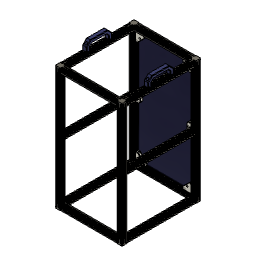
assembly (Autodesk Fusion 360 design; units mm, degrees)
Autodesk Fusion 360 part; units mm, degrees
sketch "Sketch1" plane through (0, 0, 0) normal (0, 0, 1) x (1, 0, 0) in component "2020-angle-connector"
  line L0 (10, 10) -> (-10, 10)
  line L1 (-10, 10) -> (-10, -10)
  line L2 (-10, -10) -> (10, -10)
  line L3 (10, -10) -> (10, 10)
  line L4 (10, 10) -> (-10, -10) construction
  line L5 (-10, 10) -> (10, -10) construction
  dimension "d1" = 20
  dimension "d2" = 20
  constraint horizontal L0
  constraint perpendicular L0 L1
  constraint parallel L0 L2
  constraint parallel L1 L3
  constraint coincident L4 origin
  constraint coincident L5 origin
  measures "d1" distance of L1.end L2.end
  measures "d2" distance of L0.end L1.end
extrude "Extrude1" add sketch "Sketch1" along normal blind 5 makes body 1 in component "2020-angle-connector"
fillet "Fillet1" radius 1.5 4 edges at (10, -10, 2.5) (-10, -10, 2.5) (10, 10, 2.5) (-10, 10, 2.5) on bodies 1 in component "2020-angle-connector"
sketch "Sketch2" plane through (0, -10, 0) normal (0, -1, 0) x (1, 0, 0) in component "2020-angle-connector"
  line L0 (-8.5, 5) -> (-8.5, 0)
  line L1 (-8.5, 0) -> (8.5, 0)
  line L2 (8.5, 0) -> (8.5, 5)
  line L3 (8.5, 5) -> (-8.5, 5)
  line L4 (-3, 5) -> (3, 5)
  line L5 (3, 5) -> (5, 3)
  line L6 (5, 3) -> (5, 1.5)
  line L7 (5, 1.5) -> (3, 1.5)
  line L8 (3, 1.5) -> (3, 0)
  line L9 (3, 0) -> (-3, 0)
  line L10 (-3, 0) -> (-3, 1.5)
  line L11 (-3, 1.5) -> (-5, 1.5)
  line L12 (-5, 1.5) -> (-5, 3)
  line L13 (-5, 3) -> (-3, 5)
  dimension "d7" = 10
  dimension "d8" = 6
  dimension "d9" = 135
  dimension "d11" = 1.5
  dimension "d12" = 6
  constraint parallel L3 L4
  constraint perpendicular L4 L6
  constraint perpendicular L6 L7
  constraint coincident L1 L8.end
  constraint perpendicular L1 L8
  constraint coincident L1 L9.end
  constraint perpendicular L9 L10
  constraint perpendicular L10 L11
  constraint perpendicular L11 L12
  constraint midpoint origin L9
  constraint midpoint L3 L4
  constraint equal L5 L13
  constraint equal L6 L12
  constraint equal L7 L11
  constraint equal L8 L10
  measures "d7" distance of L6 L12
  measures "d8" distance of L8 L10
  measures "d9" angle of L12 L13
  measures "d11" distance of L9.end L11
  measures "d12" distance of L4.start L4.end
extrude "Extrude2" add sketch "Sketch2" along normal blind 15.5 contours L1 L3 L4 L5 L6 L7 L8 L9 L10 L11 L12 L13 bodies 1 in component "2020-angle-connector"
pattern_circular "C-Pattern1" count 2 over 90 about axis through (0, 0, 1.75) along (0, 0, 1) of "Extrude2" in component "2020-angle-connector"
sketch "Sketch3" plane through (0, 0, 5) normal (0, 0, 1) x (-1, 0, 0) in component "2020-angle-connector"
  arc A0 (8.5, -10) -> (10, -8.5) centre (8.5, -8.5) ccw
  line L0 (10, -8.5) -> (10, 8.5)
  arc A1 (10, 8.5) -> (8.5, 10) centre (8.5, 8.5) ccw
  line L1 (8.5, 10) -> (3, 10)
  line L2 (3, 10) -> (3, 25.5)
  line L3 (3, 25.5) -> (-3, 25.5)
  line L4 (-3, 25.5) -> (-3, 10)
  line L5 (-3, 10) -> (-8.5, 10)
  arc A2 (-8.5, 10) -> (-10, 8.5) centre (-8.5, 8.5) ccw
  line L6 (-10, 8.5) -> (-10, 3)
  line L7 (-10, 3) -> (-25.5, 3)
  line L8 (-25.5, 3) -> (-25.5, -3)
  line L9 (-25.5, -3) -> (-10, -3)
  line L10 (-10, -3) -> (-10, -8.5)
  arc A3 (-10, -8.5) -> (-8.5, -10) centre (-8.5, -8.5) ccw
  line L11 (-8.5, -10) -> (8.5, -10)
  line L12 (10, -3) -> (10, 3)
  line L13 (10, 3) -> (8.5, 3)
  line L14 (8.5, 3) -> (8.5, 5)
  line L15 (8.5, 5) -> (7, 5)
  line L16 (7, 5) -> (5, 3)
  line L17 (5, 3) -> (5, -3)
  line L18 (5, -3) -> (7, -5)
  line L19 (7, -5) -> (8.5, -5)
  line L20 (8.5, -5) -> (8.5, -3)
  line L21 (8.5, -3) -> (10, -3)
  line L22 (5, 0) -> (10, 0) construction
  dimension "d17" = 6
  dimension "d18" = 10
  dimension "d19" = 1.5
  dimension "d20" = 5
  dimension "d21" = 6
  constraint coincident L0 L12.start
  constraint coincident L0 L12.end
  constraint perpendicular L0 L13
  constraint perpendicular L13 L14
  constraint perpendicular L14 L15
  constraint perpendicular L15 L17
  constraint perpendicular L16 L18
  constraint perpendicular L17 L19
  constraint perpendicular L19 L20
  constraint horizontal L21
  constraint equal L13 L21
  constraint equal L14 L20
  constraint equal L15 L19
  constraint equal L16 L18
  constraint midpoint L17 L22.start
  constraint midpoint L12 L22.end
  constraint midpoint L0 L12
  measures "d17" distance of L12.start L12.end
  measures "d18" distance of L15 L19
  measures "d19" distance of L12.start L20.end
  measures "d20" distance of L12 L17
  measures "d21" distance of L16.end L17.end
extrude "Extrude3" add sketch "Sketch3" along normal blind 15.5 contours L0 L12 L13 L14 L15 L16 L17 L18 L19 L20 L21 bodies 1 in component "2020-angle-connector"
pattern_circular "C-Pattern2" count 2 over 90 about axis through (0, 0, 1.75) along (0, 0, -1) of "Extrude3" in component "2020-angle-connector"
sketch "Sketch1 (2)" plane through (0, 0, 0) normal (0, 0, 1) x (1, 0, 0) in component "2020-profile-222,25"
  line L0 (-4.5, 0) -> (-4.5, 3.4393)
  line L1 (-7.0607, 6) -> (-8.5, 6)
  line L2 (-8.5, 6) -> (-8.5, 3)
  line L3 (-8.5, 3) -> (-10, 3)
  line L4 (-10, 3) -> (-10, 8.5)
  arc A0 (-8.5, 10) -> (-10, 8.5) centre (-8.5, 8.5) ccw
  line L5 (-8.5, 10) -> (-3, 10)
  line L6 (-3, 10) -> (-3, 8.5)
  line L7 (-3, 8.5) -> (-6, 8.5)
  line L8 (-6, 8.5) -> (-6, 7.0607)
  line L9 (-3.4393, 4.5) -> (0, 4.5)
  line L10 (0, 4.5) -> (0, 0)
  line L11 (0, 0) -> (-4.5, 0)
  line L12 (-7.0607, 6) -> (-4.5, 3.4393)
  line L13 (-6, 7.0607) -> (-3.4393, 4.5)
  circle A1 centre (0, 0) radius 2.75
  dimension "d26" = 10
  dimension "d27" = 1.5
  dimension "d28" = 4
  dimension "d29" = 5.5
  dimension "d30" = 10
  dimension "d31" = 6
  dimension "d33" = 1.5
  dimension "d34" = 3
  dimension "d35" = 5.5
  constraint vertical L0
  constraint perpendicular L0 L1
  constraint perpendicular L1 L2
  constraint perpendicular L0 L3
  constraint perpendicular L3 L4
  constraint tangent L4 A0
  constraint tangent A0 L5
  constraint perpendicular L4 L5
  constraint perpendicular L3 L6
  constraint perpendicular L6 L7
  constraint perpendicular L7 L8
  constraint perpendicular L8 L9
  constraint equal L1 L8
  constraint equal L2 L7
  constraint equal L3 L6
  constraint equal L4 L5
  constraint equal L0 L9
  constraint coincident L10.end L11.start
  constraint perpendicular L9 L10
  constraint horizontal L11
  constraint parallel L12 L13
  constraint equal L10 L11
  measures "d26" distance of L4 L10
  measures "d27" radius of A0
  measures "d28" distance of L0 L2
  measures "d29" distance of L0 L4
  measures "d30" distance of L10.end L5
  measures "d31" distance of L1 L11
  measures "d33" distance of L12 L13
  measures "d34" distance of L3 L11
  measures "d35" diameter of A1
extrude "Extrude1'" add sketch "Sketch1 (2)" along normal mid plane 222.25 separate body contours L0 L1 L2 L3 L4 A0 L5 L6 L7 L8 L9 L10 L11 L12 L13 A1 makes body 2 in component "2020-profile-222,25"
fillet "Fillet1'" radius 0.5 3 edges at (-8.5, 6, 0) (-7.0607, 6, 0) (-4.5, 3.4393, 0) on bodies 2 in component "2020-profile-222,25"
fillet "Fillet2" radius 0.25 4 edges at (-8.5, 3, 0) (-10, 3, 0) (-3, 10, 0) (-3, 8.5, 0) on bodies 2 in component "2020-profile-222,25"
fillet "Fillet3" radius 0.5 2 edges at (-6, 7.0607, 0) (-3.4393, 4.5, 0) on bodies 2 in component "2020-profile-222,25"
mirror "Mirror1" about plane through (0, 0, 0) normal (1, 0, 0) of bodies 2 merged in component "2020-profile-222,25"
mirror "Mirror2" about plane through (0, 0, 0) normal (0, 1, 0) of bodies 2 merged in component "2020-profile-222,25"
sketch "Sketch1 (3)" plane through (0, 0, 0) normal (0, 0, 1) x (1, 0, 0) in component "2020-profile-476"
  line L0 (-4.5, 0) -> (-4.5, 3.4393)
  line L1 (-7.0607, 6) -> (-8.5, 6)
  line L2 (-8.5, 6) -> (-8.5, 3)
  line L3 (-8.5, 3) -> (-10, 3)
  line L4 (-10, 3) -> (-10, 8.5)
  arc A0 (-8.5, 10) -> (-10, 8.5) centre (-8.5, 8.5) ccw
  line L5 (-8.5, 10) -> (-3, 10)
  line L6 (-3, 10) -> (-3, 8.5)
  line L7 (-3, 8.5) -> (-6, 8.5)
  line L8 (-6, 8.5) -> (-6, 7.0607)
  line L9 (-3.4393, 4.5) -> (0, 4.5)
  line L10 (0, 4.5) -> (0, 0)
  line L11 (0, 0) -> (-4.5, 0)
  line L12 (-7.0607, 6) -> (-4.5, 3.4393)
  line L13 (-6, 7.0607) -> (-3.4393, 4.5)
  circle A1 centre (0, 0) radius 2.75
  dimension "d26_1" = 10
  dimension "d27_1" = 1.5
  dimension "d28_1" = 4
  dimension "d29_1" = 5.5
  dimension "d30_1" = 10
  dimension "d31_1" = 6
  dimension "d33_1" = 1.5
  dimension "d34_1" = 3
  dimension "d35_1" = 5.5
  constraint vertical L0
  constraint perpendicular L0 L1
  constraint perpendicular L1 L2
  constraint perpendicular L0 L3
  constraint perpendicular L3 L4
  constraint tangent L4 A0
  constraint tangent A0 L5
  constraint perpendicular L4 L5
  constraint perpendicular L3 L6
  constraint perpendicular L6 L7
  constraint perpendicular L7 L8
  constraint perpendicular L8 L9
  constraint equal L1 L8
  constraint equal L2 L7
  constraint equal L3 L6
  constraint equal L4 L5
  constraint equal L0 L9
  constraint coincident L10.end L11.start
  constraint perpendicular L9 L10
  constraint horizontal L11
  constraint parallel L12 L13
  constraint equal L10 L11
  measures "d26_1" distance of L4 L10
  measures "d27_1" radius of A0
  measures "d28_1" distance of L0 L2
  measures "d29_1" distance of L0 L4
  measures "d30_1" distance of L10.end L5
  measures "d31_1" distance of L1 L11
  measures "d33_1" distance of L12 L13
  measures "d34_1" distance of L3 L11
  measures "d35_1" diameter of A1
extrude "Extrude1''" add sketch "Sketch1 (3)" along normal blind 476 separate body contours L0 L1 L2 L3 L4 A0 L5 L6 L7 L8 L9 L10 L11 L12 L13 A1 makes body 3 in component "2020-profile-476"
fillet "Fillet1''" radius 0.5 3 edges at (-8.5, 6, 238) (-7.0607, 6, 238) (-4.5, 3.4393, 238) on bodies 3 in component "2020-profile-476"
fillet "Fillet2'" radius 0.25 4 edges at (-8.5, 3, 238) (-10, 3, 238) (-3, 10, 238) (-3, 8.5, 238) on bodies 3 in component "2020-profile-476"
fillet "Fillet3'" radius 0.5 2 edges at (-6, 7.0607, 238) (-3.4393, 4.5, 238) on bodies 3 in component "2020-profile-476"
mirror "Mirror1'" about plane through (0, 0, 0) normal (1, 0, 0) of bodies 3 merged in component "2020-profile-476"
mirror "Mirror2'" about plane through (0, 0, 0) normal (0, 1, 0) of bodies 3 merged in component "2020-profile-476"
sketch "Sketch1 (4)" plane through (0, 0, 0) normal (0, 0, 1) x (1, 0, 0) in component "2020-profile-270"
  line L0 (-4.5, 0) -> (-4.5, 3.4393)
  line L1 (-7.0607, 6) -> (-8.5, 6)
  line L2 (-8.5, 6) -> (-8.5, 3)
  line L3 (-8.5, 3) -> (-10, 3)
  line L4 (-10, 3) -> (-10, 8.5)
  arc A0 (-8.5, 10) -> (-10, 8.5) centre (-8.5, 8.5) ccw
  line L5 (-8.5, 10) -> (-3, 10)
  line L6 (-3, 10) -> (-3, 8.5)
  line L7 (-3, 8.5) -> (-6, 8.5)
  line L8 (-6, 8.5) -> (-6, 7.0607)
  line L9 (-3.4393, 4.5) -> (0, 4.5)
  line L10 (0, 4.5) -> (0, 0)
  line L11 (0, 0) -> (-4.5, 0)
  line L12 (-7.0607, 6) -> (-4.5, 3.4393)
  line L13 (-6, 7.0607) -> (-3.4393, 4.5)
  circle A1 centre (0, 0) radius 2.75
  dimension "d26_2" = 10
  dimension "d27_2" = 1.5
  dimension "d28_2" = 4
  dimension "d29_2" = 5.5
  dimension "d30_2" = 10
  dimension "d31_2" = 6
  dimension "d33_2" = 1.5
  dimension "d34_2" = 3
  dimension "d35_2" = 5.5
  constraint vertical L0
  constraint perpendicular L0 L1
  constraint perpendicular L1 L2
  constraint perpendicular L0 L3
  constraint perpendicular L3 L4
  constraint tangent L4 A0
  constraint tangent A0 L5
  constraint perpendicular L4 L5
  constraint perpendicular L3 L6
  constraint perpendicular L6 L7
  constraint perpendicular L7 L8
  constraint perpendicular L8 L9
  constraint equal L1 L8
  constraint equal L2 L7
  constraint equal L3 L6
  constraint equal L4 L5
  constraint equal L0 L9
  constraint coincident L10.end L11.start
  constraint perpendicular L9 L10
  constraint horizontal L11
  constraint parallel L12 L13
  constraint equal L10 L11
  measures "d26_2" distance of L4 L10
  measures "d27_2" radius of A0
  measures "d28_2" distance of L0 L2
  measures "d29_2" distance of L0 L4
  measures "d30_2" distance of L10.end L5
  measures "d31_2" distance of L1 L11
  measures "d33_2" distance of L12 L13
  measures "d34_2" distance of L3 L11
  measures "d35_2" diameter of A1
extrude "Extrude1'''" add sketch "Sketch1 (4)" along normal blind 270 separate body contours L0 L1 L2 L3 L4 A0 L5 L6 L7 L8 L9 L10 L11 L12 L13 A1 makes body 4 in component "2020-profile-270"
fillet "Fillet1'''" radius 0.5 3 edges at (-8.5, 6, 135) (-7.0607, 6, 135) (-4.5, 3.4393, 135) on bodies 4 in component "2020-profile-270"
fillet "Fillet2''" radius 0.25 4 edges at (-8.5, 3, 135) (-10, 3, 135) (-3, 10, 135) (-3, 8.5, 135) on bodies 4 in component "2020-profile-270"
fillet "Fillet3''" radius 0.5 2 edges at (-6, 7.0607, 135) (-3.4393, 4.5, 135) on bodies 4 in component "2020-profile-270"
mirror "Mirror1''" about plane through (0, 0, 0) normal (1, 0, 0) of bodies 4 merged in component "2020-profile-270"
mirror "Mirror2''" about plane through (0, 0, 0) normal (0, 1, 0) of bodies 4 merged in component "2020-profile-270"
sketch "Sketch1 (5)" plane through (0, 0, 0) normal (1, 0, 0) x (0, 1, 0) in component "handle"
  line L0 (50, 0) -> (38, 0)
  line L1 (50, 0) -> (50, 17.8579)
  line L2 (50, 17.8579) -> (33.8579, 34)
  line L3 (33.8579, 34) -> (0, 34)
  line L4 (0, 34) -> (0, 22)
  line L5 (0, 22) -> (28.8873, 22)
  line L6 (28.8873, 22) -> (38, 12.8873)
  line L7 (38, 12.8873) -> (38, 0)
  line L8 (33.4437, 17.4437) -> (41.9289, 25.9289) construction
  dimension "d244" = 12
  dimension "d245" = 45
  dimension "d247" = 22
  dimension "d248" = 50
  constraint horizontal L0
  constraint perpendicular L0 L1
  constraint perpendicular L1 L3
  constraint perpendicular L3 L4
  constraint perpendicular L4 L5
  constraint vertical L7
  constraint parallel L2 L6
  constraint midpoint L6 L8.start
  constraint midpoint L2 L8.end
  constraint equal L0 L8
  constraint equal L0 L4
  constraint collinear origin L0.start L0.end
  constraint collinear origin L3.end L4.end
  constraint equal L6 L7
  measures "d244" distance of L0.start L0.end
  measures "d245" angle of L1 L2
  measures "d247" distance of origin L5
  measures "d248" distance of origin L0.start
extrude "Extrude1''''" add sketch "Sketch1 (5)" along normal mid plane 17 separate body makes body 5 in component "handle"
mirror "Mirror1'''" about plane through (0, 0, 34) normal (0, -1, 0) of bodies 5 merged in component "handle"
sketch "Sketch2 (2)" plane through (0, 0, 0) normal (0, 0, -1) x (1, 0, 0) in component "handle"
  line L0 (-8.5, -50) -> (8.5, -50)
  line L1 (8.5, -50) -> (8.5, -38)
  line L2 (8.5, -38) -> (-8.5, -38)
  line L3 (-8.5, -38) -> (-8.5, -50)
  line L4 (8.5, 50) -> (-8.5, 50)
  line L5 (-8.5, 50) -> (-8.5, 38)
  line L6 (-8.5, 38) -> (8.5, 38)
  line L7 (8.5, 38) -> (8.5, 50)
  line L8 (8.5, -50) -> (-8.5, -38) construction
  line L9 (8.5, 38) -> (-8.5, 50) construction
  circle A0 centre (0, -44) radius 2.1
  circle A1 centre (0, 44) radius 2.1
  circle A2 centre (0, -44) radius 3.75
  circle A3 centre (0, 44) radius 3.75
  line L10 (0, -44) -> (0, 44) construction
  dimension "d253" = 4.2
  dimension "d254" = 7.5
  constraint coincident L0.end L1.start
  constraint coincident L2.end L3.start
  constraint coincident L6.end L7.start
  constraint coincident L4.end L5.start
  constraint midpoint L8 A0.centre
  constraint midpoint L9 A1.centre
  constraint equal A0 A1
  constraint concentric A0 A2
  constraint concentric A1 A3
  constraint equal A2 A3
  constraint coincident A0.centre A2.centre
  constraint coincident A1.centre A3.centre
  measures "d253" diameter of A0
  measures "d254" diameter of A2
extrude "Extrude2'" cut sketch "Sketch2 (2)" against normal blind 45 contours A0 | A1 bodies 5 in component "handle"
extrude "Extrude3'" cut sketch "Sketch2 (2)" along normal blind 26.5 from surface at -40 contours A2 | A3 bodies 5 in component "handle"
fillet "Fillet1''''" radius 2 5 edges at (8.5, -38, 6.4437) (8.5, -33.4437, 17.4437) (8.5, 0, 22) (8.5, 33.4437, 17.4437) (8.5, 38, 6.4437) on bodies 5 in component "handle"
fillet "Fillet1''''" radius 2 5 edges at (8.5, -50, 8.9289) (8.5, -41.9289, 25.9289) (8.5, 0, 34) (8.5, 41.9289, 25.9289) (8.5, 50, 8.9289) on bodies 5 in component "handle"
fillet "Fillet1''''" radius 2 5 edges at (-8.5, 50, 8.9289) (-8.5, 41.9289, 25.9289) (-8.5, 0, 34) (-8.5, -41.9289, 25.9289) (-8.5, -50, 8.9289) on bodies 5 in component "handle"
fillet "Fillet1''''" radius 2 5 edges at (-8.5, -38, 6.4437) (-8.5, -33.4437, 17.4437) (-8.5, 0, 22) (-8.5, 33.4437, 17.4437) (-8.5, 38, 6.4437) on bodies 5 in component "handle"
sketch "Sketch1 (6)" plane through (0, 0, 0) normal (0, 1, 0) x (1, 0, 0) in component "corner-support"
  line L0 (0, 0) -> (45, 0)
  line L1 (0, 0) -> (0, -45)
  line L2 (0, -45) -> (45, 0)
  dimension "d281" = 45
  dimension "d361" = 63.6396
  constraint coincident L0.start L1.start
  constraint horizontal L0
  constraint perpendicular L0 L1
  constraint equal L0 L1
  measures "d281" distance of L0.start L1.end
  measures "d361" distance of L0.end L1.end
extrude "Extrude1'''''" add sketch "Sketch1 (6)" along normal mid plane 14 separate body makes body 6 in component "corner-support"
sketch "Sketch2 (3)" plane through (0, 0, 0) normal (-1, 0, 0) x (0, -1, 0) in component "corner-support"
  line L0 (7, 45) -> (-7, 45)
  line L1 (-7, 45) -> (-7, 0)
  line L2 (-7, 0) -> (7, 0)
  line L3 (7, 0) -> (7, 45)
  circle A0 centre (1.5, 30) radius 2.15
  line L4 (1.5, 30) -> (1.5, 45)
  circle A1 centre (1.5, 30) radius 3.75
  dimension "d284" = 4.3
  dimension "d285" = 15
  dimension "d286" = 7.5
  dimension "d299" = 8.5
  constraint coincident A0.centre L4.start
  constraint perpendicular L0 L4
  constraint concentric A0 A1
  constraint coincident L0 L4.end
  measures "d284" diameter of A0
  measures "d285" distance of A0.centre L4.end
  measures "d286" diameter of A1
  measures "d299" distance of L1 L4
extrude "Extrude2''" cut sketch "Sketch2 (3)" against normal blind 20 contours A0 bodies 6 in component "corner-support"
extrude "Extrude3''" cut sketch "Sketch2 (3)" along normal blind 14 from surface at -20 contours A1 bodies 6 in component "corner-support"
ref_plane "WorkPlane1" through (0, 0, 0) normal (-0.707107, 0, 0.707107) x (0, -1, 0) in component "corner-support"
mirror "Mirror1''''" about plane through (0, 0, 0) normal (-0.707107, 0, 0.707107) of "Extrude2''", "Extrude3''" in component "corner-support"
sketch "Sketch3 (2)" plane through (0, 7, 0) normal (0, 1, 0) x (-1, 0, 0) in component "corner-support"
  line L0 (0, 0) -> (0, 45)
  line L1 (0, 45) -> (-45, 0)
  line L2 (-45, 0) -> (0, 0)
  line L3 (-9, 36) -> (0, 36)
  line L4 (-36, 0) -> (-36, 9)
  point P0 (0, 45)
  dimension "d295" = 9
  dimension "d298" = 9
  constraint coincident L1 L3.start
  constraint coincident L0 L3.end
  constraint perpendicular L0 L3
  constraint coincident L2 L4.start
  constraint coincident L1 L4.end
  constraint perpendicular L2 L4
  measures "d295" distance of L3.end P0
  measures "d298" distance of L1.end L4.start
extrude "Extrude4" cut sketch "Sketch3 (2)" against normal blind 14 contours L0 L1 L3 | L1 L2 L4 bodies 6 in component "corner-support"
sketch "Sketch4" plane through (0, -7, 0) normal (0, -1, 0) x (1, 0, 0) in component "corner-support"
  line L0 (9, 36) -> (0, 36)
  line L1 (0, 36) -> (0, 0)
  line L2 (0, 0) -> (36, 0)
  line L3 (36, 0) -> (36, 9)
  line L4 (36, 9) -> (9, 36)
  line L5 (26, 0) -> (26, 4.8579)
  line L6 (4.8579, 26) -> (0, 26)
  circle A0 centre (17.9038, 17.9038) radius 3.2
  line L7 (8.3579, 22.5) -> (8.3579, 18.2574)
  line L8 (8.3579, 18.2574) -> (18.2574, 8.3579)
  line L9 (18.2574, 8.3579) -> (22.5, 8.3579)
  line L10 (26, 4.8579) -> (22.5, 8.3579)
  line L11 (8.3579, 22.5) -> (4.8579, 26)
  line L12 (13.3076, 13.3076) -> (22.5, 22.5) construction
  dimension "d306" = 6.4
  dimension "d307" = 13
  dimension "d308" = 14
  constraint coincident L7.start L10
  constraint vertical L7
  constraint parallel L8 L10
  constraint horizontal L9
  constraint collinear L10 L11
  constraint midpoint L8 L12.start
  constraint midpoint L4 L12.end
  constraint perpendicular L4 L12
  constraint midpoint A0.centre L12
  measures "d306" diameter of A0
  measures "d307" distance of L12.start L12.end
  measures "d308" distance of L7.end L8.end
extrude "Extrude5" add sketch "Sketch4" along normal blind 3 contours L1 L2 L5 L6 L7 L8 L9 L10 L11 bodies 6 in component "corner-support"
extrude "Extrude6" cut sketch "Sketch4" against normal blind 10.5 contours A0 bodies 6 in component "corner-support"
extrude "Extrude7" cut 1 faces at (15, 7, 15) along direction (0, -1, 0) blind 3 on bodies 6 bodies 6 in component "corner-support"
chamfer "Chamfer1" distance 0.5 angle 45 1 edges at (14.9204, -7, 19.061) on bodies 6 in component "corner-support"
chamfer "Chamfer2" distance 0.5 angle 45 2 edges at (0, 0.5045, 30.7775) (29.2225, 0.5045, 0) on bodies 6 in component "corner-support"
sketch "Sketch6" plane through (0, 0, 0) normal (0, 1, 0) x (1, 0, 0) in component "corner-support"
  line L0 (0, -36) -> (0, 0) construction
  line L1 (0, 0) -> (36, 0) construction
  line L2 (0, -36) -> (0, 0)
  line L3 (0, 0) -> (36, 0)
  constraint coincident L0.start L2.start
  constraint coincident L0.end L1.start
  constraint coincident L1.end L3.end
fillet "Fillet2'''" radius 1 1 faces at (15, 4, 15) on bodies 6 in component "corner-support"
fillet "Fillet2'''" radius 2 3 edges at (0, -3, 0) (0, -1.5, 36) (36, -1.5, 0) on bodies 6 in component "corner-support"
fillet "Fillet2'''" radius 1 2 edges at (0, -10, 13) (13, -10, 0) on bodies 6 in component "corner-support"
fillet "Fillet2'''" radius 0.5 7 edges at (2.4289, -10, 26) (6.6079, -10, 24.25) (8.3579, -10, 20.3787) (13.3076, -10, 13.3076) (20.3787, -10, 8.3579) (24.25, -10, 6.6079) (26, -10, 2.4289) on bodies 6 in component "corner-support"
fillet "Fillet2'''" radius 1 4 edges at (0, -7, 31) (0, -8.5, 26) (26, -8.5, 0) (31, -7, 0) on bodies 6 in component "corner-support"
fillet "Fillet2'''" radius 1 3 edges at (4.5, -7, 36) (22.5, -7, 22.5) (36, -7, 4.5) on bodies 6 in component "corner-support"
fillet "Fillet2'''" radius 2 2 edges at (9, -1.5, 36) (36, -1.5, 9) on bodies 6 in component "corner-support"
sketch "Sketch1 (7)" plane through (0, 0, 0) normal (0, 1, 0) x (1, 0, 0) in component "center-support"
  line L0 (0, 18) -> (0, -18)
  line L1 (-13.636, -18) -> (-20, -11.636)
  line L2 (-20, -11.636) -> (-20, 11.636)
  line L3 (-20, 11.636) -> (-13.636, 18)
  line L4 (-13.636, 18) -> (0, 18)
  line L5 (-20, 0) -> (0, 0) construction
  circle A0 centre (-13.5, 0) radius 3.2
  line L6 (-7, -7) -> (-7, 7)
  line L7 (-10, -10) -> (-10, -15)
  line L8 (-7, 7) -> (-10, 10)
  line L9 (-10, 10) -> (-10, 15)
  line L10 (-10, 15) -> (-7, 18)
  line L11 (-10, -15) -> (-7, -18)
  line L12 (-7, -7) -> (-10, -10)
  line L13 (0, -18) -> (-13.636, -18)
  point P0 (-7, 0)
  dimension "d360" = 135
  dimension "d362" = 20
  dimension "d364" = 6.4
  dimension "d365" = 6.5
  dimension "d366" = 6.5
  dimension "d367" = 14
  dimension "d368" = 10
  dimension "d371" = 5
  dimension "d373" = 135
  dimension "d374" = 135
  dimension "d376" = 135
  dimension "d377" = 135
  dimension "d379" = 9
  constraint vertical L0
  constraint perpendicular L1 L3
  constraint horizontal L4
  constraint midpoint L2 L5.start
  constraint coincident L5.end origin
  constraint horizontal L5
  constraint equal L1 L3
  constraint midpoint L5.end L0
  constraint coincident L5 A0.centre
  constraint perpendicular L5 L6
  constraint midpoint L6 P0
  constraint coincident L5 P0
  constraint parallel L6 L7
  constraint equal L7 L9
  constraint vertical L9
  constraint collinear L7 L9
  constraint coincident L4 L10.end
  constraint vertical L6.start L11.end
  constraint coincident L11.end L13
  measures "d360" angle of L1 L2
  measures "d362" distance of L0 L2
  measures "d364" diameter of A0
  measures "d365" distance of L5.start A0.centre
  measures "d366" distance of A0.centre L6
  measures "d367" distance of L6.start L6.end
  measures "d368" distance of L2 L7
  measures "d371" distance of L7.start L7.end
  measures "d373" angle of L9 L10
  measures "d374" angle of L7 L11
  measures "d376" angle of L7 L12
  measures "d377" angle of L8 L9
  measures "d379" distance of L1.start L1.end
extrude "Extrude1''''''" add sketch "Sketch1 (7)" along normal blind 17 separate body contours L0 L4 L6 L7 L8 L9 L10 L11 L12 L13 makes body 7 in component "center-support"
extrude "Extrude2'''" add sketch "Sketch1 (7)" along normal blind 14 contours L1 L2 L3 L4 L6 L7 L8 L9 L10 L11 L12 L13 | A0 bodies 7 in component "center-support"
extrude "Extrude3'''" cut sketch "Sketch1 (7)" against normal blind 10.5 from surface at 14 contours A0 bodies 7 in component "center-support"
chamfer "Chamfer1'" distance 0.5 angle 45 1 edges at (-16.4834, 14, -1.1572) on bodies 7 in component "center-support"
sketch "Sketch2 (4)" plane through (0, 0, 0) normal (1, 0, 0) x (0, 1, 0) in component "center-support"
  line L0 (0, 18) -> (0, -18)
  line L1 (0, -18) -> (17, -18)
  line L2 (17, -18) -> (17, 18)
  line L3 (17, 18) -> (0, 18)
  circle A0 centre (8.5, 13) radius 2.15
  line L4 (8.5, 18) -> (8.5, -18) construction
  circle A1 centre (8.5, -13) radius 2.15
  circle A2 centre (8.5, -13) radius 3.75
  circle A3 centre (8.5, 13) radius 3.75
  dimension "d388" = 4.3
  dimension "d389" = 8.5
  dimension "d390" = 5
  dimension "d391" = 5
  dimension "d394" = 7.5
  constraint coincident L3 L4.start
  constraint coincident L1 L4.end
  constraint perpendicular L1 L4
  constraint coincident A0.centre L4
  constraint coincident L4 A1.centre
  constraint equal A0 A1
  constraint concentric A1 A2
  constraint concentric A0 A3
  constraint equal A2 A3
  measures "d388" diameter of A0
  measures "d389" distance of L0 L4
  measures "d390" distance of A0.centre L4.start
  measures "d391" distance of L4.end A1.centre
  measures "d394" diameter of A2
extrude "Extrude4'" cut sketch "Sketch2 (4)" against normal blind 23 contours A0 | A1 bodies 7 in component "center-support"
extrude "Extrude5'" cut sketch "Sketch2 (4)" along normal blind 20 from surface at -30 contours A2 | A3 bodies 7 in component "center-support"
extrude "Extrude6'" cut 1 faces at (-6.6667, 0, -3.8787) along direction (0, 1, 0) blind 3 on bodies 7 bodies 7 in component "center-support"
chamfer "Chamfer2'" distance 0.5 angle 45 2 edges at (0, 6.4955, 13.7775) (0, 6.4955, -12.2225) on bodies 7 in component "center-support"
fillet "Fillet1'''''" radius 2 8 edges at (0, 10, 18) (0, 10, -18) (-13.636, 8.5, 18) (-20, 12.9966, 11.636) (-20, 4.0034, 11.636) (-20, 4.0034, -11.636) (-20, 12.9966, -11.636) (-13.636, 8.5, -18) on bodies 7 in component "center-support"
fillet "Fillet1'''''" radius 1 8 edges at (-10.318, 14, 18) (-16.818, 14, 14.818) (-20, 14, 0) (-16.818, 14, -14.818) (-10.318, 14, -18) (-3.5, 17, 18) (-3.5, 17, -18) (0, 17, 0) 1 faces at (-6.6667, 3, -3.8787) on bodies 7 in component "center-support"
fillet "Fillet1'''''" radius 0.5 7 edges at (-8.5, 17, 16.5) (-10, 17, 12.5) (-8.5, 17, 8.5) (-7, 17, 0) (-8.5, 17, -8.5) (-10, 17, -12.5) (-8.5, 17, -16.5) on bodies 7 in component "center-support"
fillet "Fillet1'''''" radius 1 2 edges at (-7, 15.5, -18) (-7, 15.5, 18) on bodies 7 in component "center-support"
fillet "Fillet2''''" radius 1 6 edges at (-10, 15.25, 15) (-9.8536, 16.8536, 14.9393) (-10, 15.25, 10) (-9.8536, 16.8536, 10.0607) (-7, 15.25, 7) (-6.8536, 16.8536, 7.0607) on bodies 7 in component "center-support"
fillet "Fillet2''''" radius 1 6 edges at (-7, 15.25, -7) (-6.8536, 16.8536, -7.0607) (-10, 15.25, -10) (-9.8536, 16.8536, -10.0607) (-10, 15.25, -15) (-9.8536, 16.8536, -14.9393) on bodies 7 in component "center-support"
fillet "Fillet4" radius 1 1 edges at (-6, 8.5, 0) on bodies 2 in component "2020-profile-222,25"
fillet "Fillet3'''" radius 1 12 edges at (4.8579, -8.25, 26) (4.7972, -9.8536, 25.8536) (8.3579, -8.25, 22.5) (8.2114, -9.8536, 22.4393) (8.3579, -8.25, 18.2574) (8.2114, -9.8536, 18.1967) (18.2574, -8.25, 8.3579) (18.1967, -9.8536, 8.2114) (26, -8.25, 4.8579) (25.8536, -9.8536, 4.7972) (22.5, -8.25, 8.3579) (22.4393, -9.8536, 8.2114) on bodies 6 in component "corner-support"
sketch "Sketch3 (3)" plane through (0, 0, 0) normal (1, 0, 0) x (0, 1, 0) in component "center-support"
  circle A0 centre (8.5, -13) radius 2.65
  circle A1 centre (8.5, 13) radius 2.65
  line L0 (16, 16) -> (4, 16)
  line L1 (4, 16) -> (4, -16)
  line L2 (4, -16) -> (16, -16)
  line L3 (16, -16) -> (16, 16)
  line L4 (8.5, 13) -> (8.5, -13) construction
  point P0 (8.5, 0)
  constraint coincident A1.centre L4.start
  constraint coincident A0.centre L4.end
  constraint midpoint L4 P0
sketch "Sketch1 (8)" plane through (0, 150.5, 0) normal (0, 1, 0) x (-1, 0, 0) in component "rear-panel-main"
  arc A0 (-102.4742, 448.0355) -> (-102.7671, 447.3284) centre (-101.7671, 447.3284) ccw
  line L0 (-102.7671, 447.3284) -> (-102.7671, 443.9142)
  arc A1 (-103.06, 443.2071) -> (-102.7671, 443.9142) centre (-103.7671, 443.9142) ccw
  line L1 (-103.06, 443.2071) -> (-105.9742, 440.2929)
  arc A2 (-106.6813, 440) -> (-105.9742, 440.2929) centre (-106.6813, 441) ccw
  line L2 (-106.6813, 440) -> (-110.125, 440)
  line L3 (-110.125, 440) -> (-110.125, 432) construction
  arc A3 (-110.125, 432) -> (-109.125, 431) centre (-109.125, 432) ccw construction
  line L4 (-109.125, 431) -> (-102.9534, 431) construction
  arc A4 (-102.9534, 431) -> (-102.2463, 431.2929) centre (-102.9534, 432) ccw construction
  line L5 (-102.2463, 431.2929) -> (-76.4179, 457.1213) construction
  arc A5 (-76.4179, 457.1213) -> (-76.125, 457.8284) centre (-77.125, 457.8284) ccw construction
  line L6 (-76.125, 457.8284) -> (-76.125, 464) construction
  arc A6 (-76.125, 464) -> (-77.125, 465) centre (-77.125, 464) ccw construction
  line L7 (-77.125, 465) -> (-85.125, 465) construction
  line L8 (-85.125, 465) -> (-85.125, 461.5563)
  arc A7 (-85.4179, 460.8492) -> (-85.125, 461.5563) centre (-86.125, 461.5563) ccw
  line L9 (-85.4179, 460.8492) -> (-88.3321, 457.935)
  arc A8 (-89.0392, 457.6421) -> (-88.3321, 457.935) centre (-89.0392, 458.6421) ccw
  line L10 (-89.0392, 457.6421) -> (-92.4534, 457.6421)
  arc A9 (-92.4534, 457.6421) -> (-93.1605, 457.3492) centre (-92.4534, 456.6421) ccw
  line L11 (-93.1605, 457.3492) -> (-102.4742, 448.0355)
  circle A10 centre (-93.2212, 448.0962) radius 3.7 construction
  arc A11 (93.1605, 457.3492) -> (92.4534, 457.6421) centre (92.4534, 456.6421) ccw
  line L12 (92.4534, 457.6421) -> (89.0392, 457.6421)
  arc A12 (88.3321, 457.935) -> (89.0392, 457.6421) centre (89.0392, 458.6421) ccw
  line L13 (88.3321, 457.935) -> (85.4179, 460.8492)
  arc A13 (85.125, 461.5563) -> (85.4179, 460.8492) centre (86.125, 461.5563) ccw
  line L14 (85.125, 461.5563) -> (85.125, 465)
  line L15 (85.125, 465) -> (77.125, 465) construction
  arc A14 (77.125, 465) -> (76.125, 464) centre (77.125, 464) ccw construction
  line L16 (76.125, 464) -> (76.125, 457.8284) construction
  arc A15 (76.125, 457.8284) -> (76.4179, 457.1213) centre (77.125, 457.8284) ccw construction
  line L17 (76.4179, 457.1213) -> (102.2463, 431.2929) construction
  arc A16 (102.2463, 431.2929) -> (102.9534, 431) centre (102.9534, 432) ccw construction
  line L18 (102.9534, 431) -> (109.125, 431) construction
  arc A17 (109.125, 431) -> (110.125, 432) centre (109.125, 432) ccw construction
  line L19 (110.125, 432) -> (110.125, 440) construction
  line L20 (110.125, 440) -> (106.6813, 440)
  arc A18 (105.9742, 440.2929) -> (106.6813, 440) centre (106.6813, 441) ccw
  line L21 (105.9742, 440.2929) -> (103.06, 443.2071)
  arc A19 (102.7671, 443.9142) -> (103.06, 443.2071) centre (103.7671, 443.9142) ccw
  line L22 (102.7671, 443.9142) -> (102.7671, 447.3284)
  arc A20 (102.7671, 447.3284) -> (102.4742, 448.0355) centre (101.7671, 447.3284) ccw
  line L23 (102.4742, 448.0355) -> (93.1605, 457.3492)
  circle A21 centre (93.2212, 448.0962) radius 3.7 construction
  arc A22 (104.125, 249.5858) -> (103.8321, 250.2929) centre (103.125, 249.5858) ccw
  line L24 (103.8321, 250.2929) -> (101.4179, 252.7071)
  arc A23 (101.125, 253.4142) -> (101.4179, 252.7071) centre (102.125, 253.4142) ccw
  line L25 (101.125, 253.4142) -> (101.125, 257.5858)
  arc A24 (101.4179, 258.2929) -> (101.125, 257.5858) centre (102.125, 257.5858) ccw
  line L26 (101.4179, 258.2929) -> (103.125, 260)
  line L27 (103.125, 260) -> (98.3174, 260) construction
  arc A25 (98.3174, 260) -> (97.6103, 259.7071) centre (98.3174, 259) ccw construction
  line L28 (97.6103, 259.7071) -> (92.4179, 254.5147) construction
  arc A26 (92.4179, 254.5147) -> (92.125, 253.8076) centre (93.125, 253.8076) ccw construction
  line L29 (92.125, 253.8076) -> (92.125, 232.1924) construction
  arc A27 (92.125, 232.1924) -> (92.4179, 231.4853) centre (93.125, 232.1924) ccw construction
  line L30 (92.4179, 231.4853) -> (97.6103, 226.2929) construction
  arc A28 (97.6103, 226.2929) -> (98.3174, 226) centre (98.3174, 227) ccw construction
  line L31 (98.3174, 226) -> (103.125, 226) construction
  line L32 (103.125, 226) -> (101.4179, 227.7071)
  arc A29 (101.125, 228.4142) -> (101.4179, 227.7071) centre (102.125, 228.4142) ccw
  line L33 (101.125, 228.4142) -> (101.125, 232.5858)
  arc A30 (101.4179, 233.2929) -> (101.125, 232.5858) centre (102.125, 232.5858) ccw
  line L34 (101.4179, 233.2929) -> (103.8321, 235.7071)
  arc A31 (103.8321, 235.7071) -> (104.125, 236.4142) centre (103.125, 236.4142) ccw
  line L35 (104.125, 236.4142) -> (104.125, 249.5858)
  circle A32 centre (97.625, 243) radius 3.7 construction
  arc A33 (-104.125, 236.4142) -> (-103.8321, 235.7071) centre (-103.125, 236.4142) ccw
  line L36 (-103.8321, 235.7071) -> (-101.4179, 233.2929)
  arc A34 (-101.125, 232.5858) -> (-101.4179, 233.2929) centre (-102.125, 232.5858) ccw
  line L37 (-101.125, 232.5858) -> (-101.125, 228.4142)
  arc A35 (-101.4179, 227.7071) -> (-101.125, 228.4142) centre (-102.125, 228.4142) ccw
  line L38 (-103.125, 226) -> (-98.3174, 226)
  arc A36 (-98.3174, 226) -> (-97.6103, 226.2929) centre (-98.3174, 227) ccw construction
  line L39 (-97.6103, 226.2929) -> (-92.4179, 231.4853) construction
  arc A37 (-92.4179, 231.4853) -> (-92.125, 232.1924) centre (-93.125, 232.1924) ccw construction
  line L40 (-92.125, 232.1924) -> (-92.125, 253.8076) construction
  arc A38 (-92.125, 253.8076) -> (-92.4179, 254.5147) centre (-93.125, 253.8076) ccw construction
  line L41 (-92.4179, 254.5147) -> (-97.6103, 259.7071) construction
  arc A39 (-97.6103, 259.7071) -> (-98.3174, 260) centre (-98.3174, 259) ccw construction
  line L42 (-98.3174, 260) -> (-103.125, 260) construction
  line L43 (-103.125, 260) -> (-101.4179, 258.2929)
  arc A40 (-101.125, 257.5858) -> (-101.4179, 258.2929) centre (-102.125, 257.5858) ccw
  line L44 (-101.125, 257.5858) -> (-101.125, 253.4142)
  arc A41 (-101.4179, 252.7071) -> (-101.125, 253.4142) centre (-102.125, 253.4142) ccw
  line L45 (-101.4179, 252.7071) -> (-103.8321, 250.2929)
  arc A42 (-103.8321, 250.2929) -> (-104.125, 249.5858) centre (-103.125, 249.5858) ccw
  line L46 (-104.125, 249.5858) -> (-104.125, 236.4142)
  circle A43 centre (-97.625, 243) radius 3.7 construction
  arc A44 (-93.1605, 28.6508) -> (-92.4534, 28.3579) centre (-92.4534, 29.3579) ccw
  line L47 (-92.4534, 28.3579) -> (-89.0392, 28.3579)
  arc A45 (-88.3321, 28.065) -> (-89.0392, 28.3579) centre (-89.0392, 27.3579) ccw
  line L48 (-88.3321, 28.065) -> (-85.4179, 25.1508)
  arc A46 (-85.125, 24.4437) -> (-85.4179, 25.1508) centre (-86.125, 24.4437) ccw
  line L49 (-85.125, 24.4437) -> (-85.125, 21)
  line L50 (-85.125, 21) -> (-77.125, 21) construction
  arc A47 (-77.125, 21) -> (-76.125, 22) centre (-77.125, 22) ccw construction
  line L51 (-76.125, 22) -> (-76.125, 28.1716) construction
  arc A48 (-76.125, 28.1716) -> (-76.4179, 28.8787) centre (-77.125, 28.1716) ccw construction
  line L52 (-76.4179, 28.8787) -> (-102.2463, 54.7071) construction
  arc A49 (-102.2463, 54.7071) -> (-102.9534, 55) centre (-102.9534, 54) ccw construction
  line L53 (-102.9534, 55) -> (-109.125, 55) construction
  arc A50 (-109.125, 55) -> (-110.125, 54) centre (-109.125, 54) ccw construction
  line L54 (-110.125, 54) -> (-110.125, 46) construction
  line L55 (-110.125, 46) -> (-106.6813, 46)
  arc A51 (-105.9742, 45.7071) -> (-106.6813, 46) centre (-106.6813, 45) ccw
  line L56 (-105.9742, 45.7071) -> (-103.06, 42.7929)
  arc A52 (-102.7671, 42.0858) -> (-103.06, 42.7929) centre (-103.7671, 42.0858) ccw
  line L57 (-102.7671, 42.0858) -> (-102.7671, 38.6716)
  arc A53 (-102.7671, 38.6716) -> (-102.4742, 37.9645) centre (-101.7671, 38.6716) ccw
  line L58 (-102.4742, 37.9645) -> (-93.1605, 28.6508)
  circle A54 centre (-93.2212, 37.9038) radius 3.7 construction
  arc A55 (102.4742, 37.9645) -> (102.7671, 38.6716) centre (101.7671, 38.6716) ccw
  line L59 (102.7671, 38.6716) -> (102.7671, 42.0858)
  arc A56 (103.06, 42.7929) -> (102.7671, 42.0858) centre (103.7671, 42.0858) ccw
  line L60 (103.06, 42.7929) -> (105.9742, 45.7071)
  arc A57 (106.6813, 46) -> (105.9742, 45.7071) centre (106.6813, 45) ccw
  line L61 (106.6813, 46) -> (110.125, 46)
  line L62 (110.125, 46) -> (110.125, 54) construction
  arc A58 (110.125, 54) -> (109.125, 55) centre (109.125, 54) ccw construction
  line L63 (109.125, 55) -> (102.9534, 55) construction
  arc A59 (102.9534, 55) -> (102.2463, 54.7071) centre (102.9534, 54) ccw construction
  line L64 (102.2463, 54.7071) -> (76.4179, 28.8787) construction
  arc A60 (76.4179, 28.8787) -> (76.125, 28.1716) centre (77.125, 28.1716) ccw construction
  line L65 (76.125, 28.1716) -> (76.125, 22) construction
  arc A61 (76.125, 22) -> (77.125, 21) centre (77.125, 22) ccw construction
  line L66 (77.125, 21) -> (85.125, 21) construction
  line L67 (85.125, 21) -> (85.125, 24.4437)
  arc A62 (85.4179, 25.1508) -> (85.125, 24.4437) centre (86.125, 24.4437) ccw
  line L68 (85.4179, 25.1508) -> (88.3321, 28.065)
  arc A63 (89.0392, 28.3579) -> (88.3321, 28.065) centre (89.0392, 27.3579) ccw
  line L69 (89.0392, 28.3579) -> (92.4534, 28.3579)
  arc A64 (92.4534, 28.3579) -> (93.1605, 28.6508) centre (92.4534, 29.3579) ccw
  line L70 (93.1605, 28.6508) -> (102.4742, 37.9645)
  circle A65 centre (93.2212, 37.9038) radius 3.7 construction
  line L71 (-101.4179, 258.2929) -> (-103.125, 260)
  line L72 (-102.7475, 259.6225) -> (-101.4179, 258.2929)
  line L73 (101.4179, 227.7071) -> (103.125, 226)
  line L74 (102.7475, 226.3775) -> (101.4179, 227.7071)
  line L75 (101.4179, 258.2929) -> (102.7475, 259.6225)
  line L76 (103.8321, 260.7071) -> (102.7475, 259.6225)
  line L77 (103.125, 260) -> (101.4179, 258.2929)
  arc A66 (104.5392, 261) -> (103.8321, 260.7071) centre (104.5392, 260) ccw
  ellipse E0 centre (104.5392, 260) end of major axis (105.5392, 260) minor radius 1 (104.5392, 261) -> (103.8321, 260.7071) ccw
  line L78 (-111.125, 20) -> (111.125, 20)
  line L79 (-111.125, 5) -> (-111.125, 481)
  line L80 (111.125, 466) -> (-111.125, 466)
  line L81 (111.125, 5) -> (111.125, 481)
  line L82 (-85.125, 465) -> (-85.125, 466)
  line L83 (-110.125, 440) -> (-111.125, 440)
  line L84 (85.125, 465) -> (85.125, 466)
  line L85 (110.125, 440) -> (111.125, 440)
  line L86 (-110.125, 46) -> (-111.125, 46)
  line L87 (-85.125, 21) -> (-85.125, 20)
  line L88 (85.125, 21) -> (85.125, 20)
  line L89 (110.125, 46) -> (111.125, 46)
  arc A67 (103.8321, 225.2929) -> (104.5392, 225) centre (104.5392, 226) ccw
  line L90 (101.4179, 227.7071) -> (103.125, 226)
  line L91 (103.125, 226) -> (103.8321, 225.2929)
  line L92 (104.5392, 225) -> (111.125, 225)
  arc A68 (-103.8321, 260.7071) -> (-104.5392, 261) centre (-104.5392, 260) ccw
  line L93 (-103.125, 260) -> (-103.8321, 260.7071)
  line L94 (-104.5392, 261) -> (-111.125, 261)
  line L95 (-103.125, 226) -> (-101.4179, 227.7071)
  line L96 (-103.8321, 225.2929) -> (-103.125, 226)
  arc A69 (-104.5392, 225) -> (-103.8321, 225.2929) centre (-104.5392, 226) ccw
  line L97 (-111.125, 225) -> (-104.5392, 225)
  circle A70 centre (-93.2212, 37.9038) radius 2.55
  circle A71 centre (93.2212, 37.9038) radius 2.55
  circle A72 centre (-97.625, 243) radius 2.55
  circle A73 centre (97.625, 243) radius 2.55
  circle A74 centre (-93.2212, 448.0962) radius 2.55
  circle A75 centre (93.2212, 448.0962) radius 2.55
  line L98 (111.125, 261) -> (104.5392, 261)
  point P0 (103.125, 226)
  dimension "d483" = 5.1
  constraint coincident L7.end L8.start
  constraint coincident L80 L82.end
  constraint perpendicular L80 L82
  constraint coincident L2.end L3.start
  constraint coincident L79 L83.end
  constraint perpendicular L79 L83
  constraint coincident L14.end L15.start
  constraint coincident L80 L84.end
  constraint perpendicular L80 L84
  constraint coincident L19.end L20.start
  constraint coincident L81 L85.end
  constraint perpendicular L81 L85
  constraint coincident L54.end L55.start
  constraint coincident L79 L86.end
  constraint perpendicular L79 L86
  constraint coincident L49.end L50.start
  constraint coincident L78 L87.end
  constraint perpendicular L50 L87
  constraint coincident L66.end L67.start
  constraint coincident L78 L88.end
  constraint perpendicular L78 L88
  constraint coincident L61.end L62.start
  constraint coincident L81 L89.end
  constraint perpendicular L81 L89
  constraint coincident A67.end L92.start
  constraint coincident L81 L92.end
  constraint tangent A67 L92
  constraint coincident A68.end L94.start
  constraint coincident L79 L94.end
  constraint tangent A68 L94
  constraint coincident L79 L97.start
  constraint coincident A69.start L97.end
  constraint horizontal L97
  constraint concentric A54 A70
  constraint concentric A65 A71
  constraint concentric A43 A72
  constraint concentric A32 A73
  constraint concentric A10 A74
  constraint concentric A21 A75
  constraint equal A74 A75
  constraint equal A73 A75
  constraint equal A72 A73
  constraint equal A71 A72
  constraint equal A70 A71
  constraint coincident L81 L98.start
  constraint coincident A66.start L98.end
  constraint horizontal L98
  measures "d483" diameter of A70
extrude "Extrude1'''''''" add sketch "Sketch1 (8)" along normal blind 3 separate body contours A0 L0 A1 L1 A2 L2 L8 A7 L9 A8 L10 A9 L11 A11 L12 A12 L13 A13 L14 L20 A18 L21 A19 L22 A20 L23 A22 L24 A23 L25 A24 L26 L32 A29 L33 A30 L34 A31 L35 A33 L36 A34 L37 A35 L43 A40 L44 A41 L45 A42 L46 A44 L47 A45 L48 A46 L49 L55 A51 L56 A52 L57 A53 L58 A55 L59 A56 L60 A57 L61 L67 A62 L68 A63 L69 A64 L70 L71 L72 L73 L74 L75 L76 L77 A66 E0 L78 L79 L80 L81 L82 L83 L84 L85 L86 L87 L88 L89 A67 L90 L91 L92 A68 L93 L94 L95 L96 A69 L97 L98 makes body 8 in component "rear-panel-main"
component "structure" placed x (1, 0, 0) y (0, 1, 0) z (0, 0, 1) at (0, 0, 0)
component "rear-panel" placed x (1, 0, 0) y (0, 1, 0) z (0, 0, 1) at (0, 0, 0)
component "handle" placed x (1, 0, 0) y (0, 1, 0) z (0, 0, 1) at (-121.125, 0, 486)
component "handle" placed x (1, 0, 0) y (0, 1, 0) z (0, 0, 1) at (121.125, 0, 486)
component "2020-profile-270" placed x (1, 0, 0) y (0, 0, 1) z (0, -1, 0) at (-121.125, 135, 243) in component "structure"
component "2020-angle-connector" placed x (0, 1, 0) y (-1, 0, 0) z (0, 0, 1) at (-121.125, -145, 0) in component "structure"
component "2020-angle-connector" placed x (1, 0, 0) y (0, 1, 0) z (0, 0, 1) at (-121.125, 145, 0) in component "structure"
component "2020-angle-connector" placed x (-1, 0, 0) y (0, -1, 0) z (0, 0, 1) at (121.125, -145, 0) in component "structure"
component "2020-profile-222,25" placed x (0, 0, -1) y (0, 1, 0) z (1, 0, 0) at (0, -145, 10) in component "structure"
component "2020-profile-476" placed x (1, 0, 0) y (0, 1, 0) z (0, 0, 1) at (121.125, -145, 5) in component "structure"
component "2020-profile-270" placed x (1, 0, 0) y (0, 0, -1) z (0, 1, 0) at (-121.125, -135, 10) in component "structure"
component "2020-profile-270" placed x (1, 0, 0) y (0, 0, -1) z (0, 1, 0) at (121.125, -135, 10) in component "structure"
component "2020-angle-connector" placed x (0, -1, 0) y (1, 0, 0) z (0, 0, 1) at (121.125, 145, 0) in component "structure"
component "2020-profile-476" placed x (1, 0, 0) y (0, 1, 0) z (0, 0, 1) at (-121.125, -145, 5) in component "structure"
component "2020-profile-222,25" placed x (0, 0, -1) y (0, -1, 0) z (-1, 0, 0) at (0, 145, 10) in component "structure"
component "2020-profile-476" placed x (0, 1, 0) y (-1, 0, 0) z (0, 0, 1) at (121.125, 145, 5) in component "structure"
component "2020-profile-476" placed x (0, -1, 0) y (1, 0, 0) z (0, 0, 1) at (-121.125, 145, 5) in component "structure"
component "2020-angle-connector" placed x (0, 1, 0) y (1, 0, 0) z (0, 0, -1) at (121.125, -145, 486) in component "structure"
component "2020-angle-connector" placed x (1, 0, 0) y (0, -1, 0) z (0, 0, -1) at (-121.125, -145, 486) in component "structure"
component "2020-angle-connector" placed x (0, -1, 0) y (-1, 0, 0) z (0, 0, -1) at (-121.125, 145, 486) in component "structure"
component "2020-angle-connector" placed x (-1, 0, 0) y (0, 1, 0) z (0, 0, -1) at (121.125, 145, 486) in component "structure"
component "2020-profile-270" placed x (1, 0, 0) y (0, 0, 1) z (0, -1, 0) at (121.125, 135, 476) in component "structure"
component "2020-profile-270" placed x (1, 0, 0) y (0, 0, 1) z (0, -1, 0) at (-121.125, 135, 476) in component "structure"
component "2020-profile-222,25" placed x (0, 0, 1) y (0, -1, 0) z (1, 0, 0) at (0, -145, 476) in component "structure"
component "2020-profile-222,25" placed x (0, 0, 1) y (0, -1, 0) z (1, 0, 0) at (0, 145, 476) in component "structure"
component "2020-profile-270" placed x (1, 0, 0) y (0, 0, 1) z (0, -1, 0) at (121.125, 135, 243) in component "structure"
component "corner-support" placed x (-1, 0, 0) y (0, -1, 0) z (0, 0, 1) at (111.125, 143.5, 20) in component "rear-panel"
component "corner-support" placed x (1, 0, 0) y (0, -1, 0) z (0, 0, -1) at (-111.125, 143.5, 466) in component "rear-panel"
component "corner-support" placed x (0, 0, -1) y (0, -1, 0) z (-1, 0, 0) at (111.125, 143.5, 466) in component "rear-panel"
component "corner-support" placed x (0, 0, 1) y (0, -1, 0) z (1, 0, 0) at (-111.125, 143.5, 20) in component "rear-panel"
component "center-support" placed x (1, 0, 0) y (0, 1, 0) z (0, 0, 1) at (111.125, 136.5, 243) in component "rear-panel"
component "center-support" placed x (-1, 0, 0) y (0, 1, 0) z (0, 0, -1) at (-111.125, 136.5, 243) in component "rear-panel"
component "rear-panel-main" placed x (1, 0, 0) y (0, 1, 0) z (0, 0, 1) at (0, 0, 0) in component "rear-panel"
equation "d258 = 20.00 mm + 6.5 mm"
